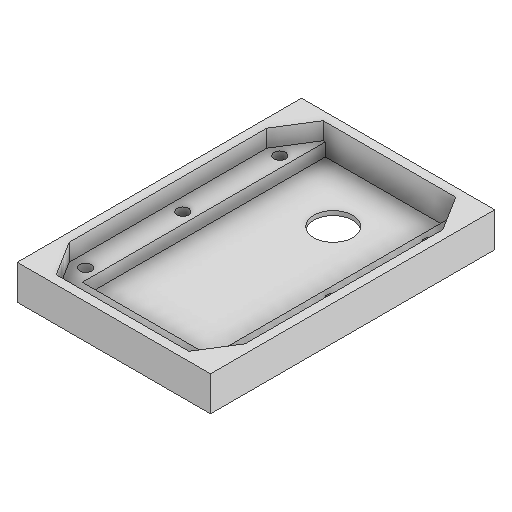
# Autodesk Inventor part: mx-64
Saved by Autodesk Inventor 2025.2 (Build 292293000, 293)
## iProperties
Created: 2025-06-17
Part Number: mx-64
Material: 일반
Document SubType Name: Modeling
Designer: joseph
Density: 1 g/cm^3
Appearance: 기본값
Author: joseph
Autodesk Inventor part; units mm, degrees
ref_plane "YZ Plane" through (0, 0, 0) normal (1, 0, 0) x (0, 1, 0)
ref_plane "XZ Plane" through (0, 0, 0) normal (0, 1, 0) x (-1, 0, 0)
ref_plane "XY Plane" through (0, 0, 0) normal (0, 0, 1) x (1, 0, 0)
sketch "스케치1" plane through (0, 0, 0) normal (0, 1, 0) x (-1, 0, 0)
  line L0 (0, 0) -> (40.6, 0)
  line L1 (40.6, 0) -> (40.6, -61.6)
  line L2 (40.6, -61.6) -> (0, -61.6)
  line L3 (0, -61.6) -> (0, 0)
  line L4 (42.6, -63.6) -> (42.6, 2)
  line L5 (42.6, 2) -> (-2, 2)
  line L6 (-2, 2) -> (-2, -63.6)
  line L7 (-2, -63.6) -> (42.6, -63.6)
  line L8 (35.6, 0) -> (40.6, -8)
  line L9 (40.6, -30.8) -> (0, -30.8) construction
  line L10 (20.3, 0) -> (20.3, -61.6) construction
  line L11 (35.6, -61.6) -> (40.6, -53.6)
  line L12 (0, 0) -> (0, -61.6)
  line L13 (5, 0) -> (0, -8)
  line L14 (5, -61.6) -> (0, -53.6)
  point P0 (0, -8)
  point P1 (5, 0)
  point P2 (40.6, -53.6)
  point P3 (0, -53.6)
  dimension "d0" = 40.6
  dimension "d1" = 61.6
  dimension "d2" = 2
  dimension "d3" = 5
  dimension "d4" = 8
  constraints: 30 end point, 6 symmetric about line, 4 midpoint, 4 parallel, 3 point on line, 2 perpendicular, 1 horizontal, 3 other
  measures "d0" distance of L1.end L2.end
  measures "d1" distance of L0.end L1.end
  measures "d2" distance between parallel lines of L1 L4
  measures "d3" distance of L8.start L0.end
  measures "d4" distance of L8.end L0.end
extrude "돌출1" add sketch "스케치1" along normal blind 7 contours L0 L13 L3 | L0 L1 L8 | L14 L2 L3 | L1 L2 L11 | L7 L6 L5 L4
sketch "스케치2" plane through (0, 0, 0) normal (0, -1, 0) x (1, 0, 0)
  line L0 (-42.6, 2) -> (2, 2) projected
  line L1 (-42.6, -63.6) -> (-42.6, 2) projected
  line L2 (2, -63.6) -> (-42.6, -63.6) projected
  line L3 (2, 2) -> (2, -63.6) projected
  line L4 (0, -53.6) -> (0, -8) projected
  line L5 (-5, -61.6) -> (0, -53.6) projected
  line L6 (-35.6, -61.6) -> (-5, -61.6) projected
  line L7 (-40.6, -53.6) -> (-35.6, -61.6) projected
  line L8 (-40.6, -8) -> (-40.6, -53.6) projected
  line L9 (-35.6, 0) -> (-40.6, -8) projected
  line L10 (-5, 0) -> (-35.6, 0) projected
  line L11 (0, -8) -> (-5, 0) projected
  point P0 (0, 0)
extrude "돌출2" add sketch "스케치2" along normal blind 1 contours L0 L3 L2 L1 | L5 L6 L7 L8 L9 L10 L11 L4
sketch "스케치3" plane through (0, 0, 0) normal (0, 1, 0) x (1, 0, 0)
  line L0 (-42.6, -2) -> (2, -2) projected
  line L1 (2, -2) -> (2, 63.6) projected
  line L2 (2, 63.6) -> (-42.6, 63.6) projected
  line L3 (-42.6, 63.6) -> (-42.6, -2) projected
  line L4 (0, 53.6) -> (0, 8) projected
  line L5 (0, 8) -> (-5, 0) projected
  line L6 (-5, 0) -> (-35.6, 0) projected
  line L7 (-35.6, 0) -> (-40.6, 8) projected
  line L8 (-40.6, 8) -> (-40.6, 53.6) projected
  line L9 (-40.6, 53.6) -> (-35.6, 61.6) projected
  line L10 (-35.6, 61.6) -> (-5, 61.6) projected
  line L11 (-5, 61.6) -> (0, 53.6) projected
  line L12 (-35.1, 61.6) -> (-5.5, 61.6)
  line L13 (-5.5, 61.6) -> (-5.5, 5.5)
  line L14 (-5.5, 5.5) -> (-35.1, 5.5)
  line L15 (-35.1, 5.5) -> (-35.1, 61.6)
  line L16 (-35.6, 61.6) -> (-5, 61.6) projected
  point P0 (0, 0)
  dimension "d9" = 5.5
  dimension "d10" = 5.5
  dimension "d11" = 5.5
  constraints: 8 end point, 2 parallel, 1 collinear, 1 horizontal, 1 perpendicular
  measures "d9" distance between parallel lines of L15 L8
  measures "d10" distance between parallel lines of L4 L13
  measures "d11" distance between parallel lines of L6 L14
extrude "돌출3" add sketch "스케치3" along normal blind 3 contours L4 L5 L6 L7 L8 L9 L10 L15 L14 L13 L11
sketch "스케치4" plane through (0, 0, 0) normal (0, 1, 0) x (1, 0, 0)
  line L0 (-5.5, 5.5) -> (-5.5, 61.6) projected
  line L1 (-35.1, 61.6) -> (-5.5, 61.6) projected
  line L2 (-35.1, 61.6) -> (-35.1, 5.5) projected
  line L3 (-35.1, 5.5) -> (-5.5, 5.5) projected
  circle A0 centre (-20.3, 48.6) radius 4.5
  point P0 (0, 0)
  dimension "d15" = 9
  dimension "d18" = 13
  constraints: 1 centre point
  measures "d15" diameter of A0
  measures "d18" distance from line of L1 A0.centre
extrude "돌출4" cut sketch "스케치4" against normal blind 7 contours A0
sketch "스케치5" plane through (0, 3, 0) normal (0, 1, 0) x (1, 0, 0)
  line L0 (-42.6, -2) -> (2, -2) projected
  line L1 (-40.6, 8) -> (-40.6, 53.6) projected
  line L2 (-35.6, 0) -> (-40.6, 8) projected
  line L3 (-5, 0) -> (-35.6, 0) projected
  line L4 (0, 8) -> (-5, 0) projected
  line L5 (0, 53.6) -> (0, 8) projected
  line L6 (-5, 61.6) -> (0, 53.6) projected
  line L7 (-5.5, 61.6) -> (-5, 61.6) projected
  line L8 (-5.5, 61.6) -> (-5.5, 5.5) projected
  line L9 (-5.5, 5.5) -> (-35.1, 5.5) projected
  line L10 (-35.1, 5.5) -> (-35.1, 61.6) projected
  line L11 (-35.6, 61.6) -> (-35.1, 61.6) projected
  line L12 (-40.6, 53.6) -> (-35.6, 61.6) projected
  line L13 (-37.6, 4.5) -> (-37.6, 58.8776) construction
  circle A0 centre (-37.6, 53.6) radius 1.35
  line L14 (2, 63.6) -> (-42.6, 63.6) construction
  circle A1 centre (-37.6, 31.2) radius 1.35
  circle A2 centre (-37.6, 8.8) radius 1.35
  line L15 (-20.3, 5.5) -> (-20.3, 61.6) construction
  line L16 (-35.6, 61.6) -> (-5, 61.6) construction
  line L17 (-5, 0) -> (0, 8)
  line L18 (-5.5, 5.5) -> (-5.5, 61.6)
  circle A3 centre (-3, 53.6) radius 1.35
  circle A4 centre (-3, 31.2) radius 1.35
  circle A5 centre (-3, 8.8) radius 1.35
  point P0 (0, 0)
  dimension "d20" = 2.7
  dimension "d21" = 10
  dimension "d24" = 22.4
  dimension "d31" = 34.6
  constraints: 8 end point, 6 centre point, 3 symmetric about line, 2 midpoint, 2 vertical, 1 point on line, 7 other
  measures "d20" diameter of A0
  measures "d21" distance from line of L14 A0.centre
  measures "d24" distance of A0.centre A1.centre
  measures "d31" distance of A3.centre A0.centre
extrude "돌출5" cut sketch "스케치5" against normal through all contours A0 | A1 | A2 | A3 | A4 | A5
